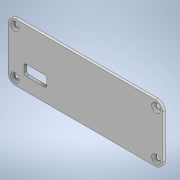
# Autodesk Inventor part: cover
Saved by Autodesk Inventor 2021 (Build 250183000, 183)
## iProperties
Created: 2025-06-25
Part Number: cover
Material: Generic
Document SubType Name: Modeling
Designer: Toby
Density: 1 g/cm^3
Appearance: Default
Author: Toby
Autodesk Inventor part; units mm, degrees
ref_plane "YZ Plane" through (0, 0, 0) normal (1, 0, 0) x (0, 1, 0)
ref_plane "XZ Plane" through (0, 0, 0) normal (0, 1, 0) x (-1, 0, 0)
ref_plane "XY Plane" through (0, 0, 0) normal (0, 0, 1) x (1, 0, 0)
sketch "Sketch1" plane through (0, 0, 0) normal (0, 0, 1) x (1, 0, 0)
  line L0 (-35.5, 13.25) -> (35.5, 13.25)
  line L1 (35.5, 13.25) -> (35.5, -13.25)
  line L2 (35.5, -13.25) -> (-35.5, -13.25)
  line L3 (-35.5, -13.25) -> (-35.5, 13.25)
  point P0 (0, 0)
  dimension "d0" = 26.5
  dimension "d1" = 71
  dimension "d2" = 35.5
  dimension "d3" = 13.25
  constraints: 8 end point, 2 parallel, 1 horizontal, 1 perpendicular
  measures "d0" distance of L2.end L0.start
  measures "d1" distance of L0.start L0.end
  measures "d2" distance from line of point (0, 0) L3
  measures "d3" distance from line of point (0, 0) L0
extrude "Extrusion1" add sketch "Sketch1" along normal blind 1.2
fillet "Fillet1" radius 3.25 4 edges at (-35.5, 13.25, 0.6) (-35.5, -13.25, 0.6) (35.5, -13.25, 0.6) (35.5, 13.25, 0.6)
sketch "Sketch2" plane through (0, 0, 1.2) normal (0, 0, 1) x (1, 0, 0)
  line L0 (32.25, 13.25) -> (-32.25, 13.25) projected
  line L1 (-35.5, 10) -> (-35.5, -10) projected
  line L2 (-32.25, -13.25) -> (32.25, -13.25) projected
  line L3 (35.5, -10) -> (35.5, 10) projected
  point P0 (0, 0)
  point P1 (-32.5, 10.25)
  point P2 (32.5, 10.25)
  point P3 (32.5, -10.25)
  point P4 (-32.5, -10.25)
  dimension "d7" = 3
  dimension "d8" = 3
  dimension "d9" = 3
  dimension "d10" = 3
  dimension "d11" = 3
  dimension "d12" = 3
  dimension "d13" = 3
  dimension "d14" = 3
  measures "d7" distance from line of L0 point (-32.5, 10.25)
  measures "d8" distance from line of L1 point (-32.5, 10.25)
  measures "d9" distance from line of L1 point (-32.5, -10.25)
  measures "d10" distance from line of L2 point (-32.5, -10.25)
  measures "d11" distance from line of L3 point (32.5, -10.25)
  measures "d12" distance from line of L2 point (32.5, -10.25)
  measures "d13" distance from line of L0 point (32.5, 10.25)
  measures "d14" distance from line of L3 point (32.5, 10.25)
hole "Hole1" at (-32.5, 10.25, 1.2) at (32.5, 10.25, 1.2) at (32.5, -10.25, 1.2) at (-32.5, -10.25, 1.2) direction (0, 0, -1) diameter 2 depth 4 tip angle 118 countersink diameter 4 countersink angle 90
sketch "Sketch3" plane through (0, 0, 1.2) normal (0, 0, 1) x (1, 0, 0)
  line L0 (-28.2, -2.25) -> (-17.8, -2.25)
  line L1 (-17.8, -2.25) -> (-17.8, -7.05)
  line L2 (-17.8, -7.05) -> (-28.2, -7.05)
  line L3 (-28.2, -7.05) -> (-28.2, -2.25)
  line L4 (-35.5, 10) -> (-35.5, -10) projected
  line L5 (-32.25, -13.25) -> (32.25, -13.25) projected
  point P0 (0, 0)
  dimension "d22" = 7.3
  dimension "d23" = 17.7
  dimension "d24" = 6.2
  dimension "d25" = 11
  constraints: 8 end point, 2 parallel, 1 horizontal, 1 perpendicular
  measures "d22" distance between parallel lines of L4 L3
  measures "d23" distance between parallel lines of L4 L1
  measures "d24" distance between parallel lines of L5 L2
  measures "d25" distance between parallel lines of L5 L0
extrude "Extrusion2" cut sketch "Sketch3" against normal blind 1.2
fillet "Fillet2" radius 1 4 edges at (-28.2, -2.25, 0.6) (-28.2, -7.05, 0.6) (-17.8, -2.25, 0.6) (-17.8, -7.05, 0.6)
sketch "Sketch4" plane through (0, 0, 0) normal (0, 0, -1) x (-1, 0, 0)
  line L0 (-29.5, 8.25) -> (29.5, 8.25)
  line L1 (29.5, 8.25) -> (29.5, 6.25)
  line L2 (29.5, 6.25) -> (-29.5, 6.25)
  line L3 (-29.5, 6.25) -> (-29.5, 8.25)
  line L4 (-35.5, -10) -> (-35.5, 10) projected
  line L5 (35.5, 10) -> (35.5, -10) projected
  line L6 (-32.25, 13.25) -> (32.25, 13.25) projected
  point P0 (0, 0)
  dimension "d29" = 6
  dimension "d30" = 6
  dimension "d31" = 5
  dimension "d32" = 2
  constraints: 8 end point, 2 parallel, 1 horizontal, 1 perpendicular
  measures "d29" distance between parallel lines of L4 L3
  measures "d30" distance between parallel lines of L5 L1
  measures "d31" distance between parallel lines of L0 L6
  measures "d32" distance between parallel lines of L2 L0
extrude "Extrusion3" add sketch "Sketch4" along normal blind 3
fillet "Fillet3" radius 1 2 edges at (0, 6.25, 0) (0, 8.25, 0)
chamfer "Chamfer1" distance 3 angle 45 2 edges at (29.5, 7.25, -3) (-29.5, 7.25, -3)
body "Solid1"
